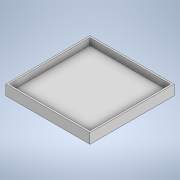
# Autodesk Inventor part: Деталь2
Saved by Autodesk Inventor 2022.4 (Build 264492010, 492A)
## iProperties
Created: 2023-02-20
Part Number: Деталь2
Material: Типовые
Document SubType Name: Modeling
Designer: artyo
Density: 1 g/cm^3
Appearance: По умолчанию
Author: artyo
Autodesk Inventor part; units mm, degrees
ref_plane "YZ Plane" through (0, 0, 0) normal (1, 0, 0) x (0, 1, 0)
ref_plane "XZ Plane" through (0, 0, 0) normal (0, 1, 0) x (-1, 0, 0)
ref_plane "XY Plane" through (0, 0, 0) normal (0, 0, 1) x (1, 0, 0)
sketch "Эскиз1" plane through (0, 0, 0) normal (0, 1, 0) x (-1, 0, 0)
  line L0 (-250, -250) -> (250, -250)
  line L1 (250, -250) -> (250, 250)
  line L2 (250, 250) -> (-250, 250)
  line L3 (-250, 250) -> (-250, -250)
  line L4 (-250, -250) -> (250, 250) construction
  line L5 (250, -250) -> (-250, 250) construction
  point P0 (0, 0)
  dimension "d0" = 500
  dimension "d1" = 500
  constraints: 12 end point, 2 midpoint, 2 parallel, 1 horizontal, 1 perpendicular
  measures "d0" distance of L2.end L1.end
  measures "d1" distance of L1.end L0.end
extrude "Выдавливание1" add sketch "Эскиз1" along normal blind 20
sketch "Эскиз2" plane through (0, 20, 0) normal (0, 1, 0) x (1, 0, 0)
  line L0 (-250, 250) -> (-250, -250) projected
  line L1 (250, 250) -> (-250, 250)
  line L2 (-250, 250) -> (-250, -250)
  line L3 (-250, -250) -> (250, -250)
  line L4 (250, -250) -> (250, 250)
  line L5 (250, 250) -> (-250, -250) construction
  line L6 (-250, 250) -> (250, -250) construction
  line L7 (240, 240) -> (-240, 240)
  line L8 (-240, 240) -> (-240, -240)
  line L9 (-240, -240) -> (240, -240)
  line L10 (240, -240) -> (240, 240)
  line L11 (240, 240) -> (-240, -240) construction
  line L12 (-240, 240) -> (240, -240) construction
  point P0 (0, 0)
  dimension "d4" = 480
  dimension "d5" = 480
  constraints: 24 end point, 4 midpoint, 4 parallel, 2 horizontal, 2 perpendicular
  measures "d4" distance of L9.end L8.end
  measures "d5" distance of L8.end L7.end
extrude "Выдавливание2" add sketch "Эскиз2" along normal blind 40
